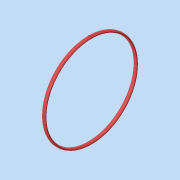
# Autodesk Inventor part: ORingA50_2.987ID_3.193OD_Compressed
Saved by Autodesk Inventor 2017 (Build 210142000, 142)
## iProperties
Created: 2016-11-20
Part Number: ORingA50_2.987ID_3.193OD_Compressed
Material: Rubber, Silicone
Document SubType Name: Modeling
Designer: techn
Density: 1.25 g/cm^3
Appearance: Smooth - Red
Author: techn
Autodesk Inventor part; units mm, degrees
ref_plane "YZ Plane" through (0, 0, 0) normal (1, 0, 0) x (0, 1, 0)
ref_plane "XZ Plane" through (0, 0, 0) normal (0, 1, 0) x (-1, 0, 0)
ref_plane "XY Plane" through (0, 0, 0) normal (0, 0, 1) x (1, 0, 0)
sketch "Sketch1" plane through (0, 0, 0) normal (0, 0, 1) x (1, 0, 0)
  line L0 (0, 41.275) -> (0, 39.243)
  ellipse E0 centre (0, 40.259) end of major axis (1.5867, 40.259) minor radius 1.016
  line L1 (0, 0) -> (-3.3795, 0)
  dimension "d2" = 39.243
  dimension "d3" = 41.275
  constraints: 4 end point, 2 vertical, 1 horizontal, 1 midpoint, 1 vertical alignment, 2 other
  measures "d2" distance of L0.end L1.start
  measures "d3" distance of L1.start L0.start
revolve "Revolution1" add sketch "Sketch1" angle 360 about axis through (0, 0, 0) along (-1, 0, 0)
body "Solid1"
